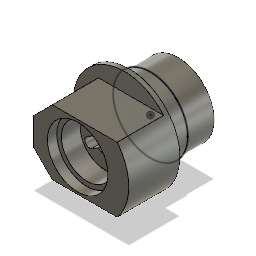
912-002_SpanDriver (Autodesk Fusion 360 design; units mm, degrees)
Autodesk Fusion 360 part; units mm, degrees
sketch "Sketch1" plane through (0, 0, 0) normal (0, 0, 1) x (1, 0, 0)
  circle A0 centre (0, 0) radius 3.875
  circle A1 centre (0, 0) radius 2.6825 construction
  circle A2 centre (0, 0) radius 2.356 construction
  line L0 (0, 2.356) -> (0, 2.6825)
  line L1 (-0.3686, 2.327) -> (-0.4196, 2.6495)
  line L2 (-0.728, 2.2407) -> (-0.8289, 2.5512)
  line L3 (-1.0696, 2.0992) -> (-1.2178, 2.3901)
  line L4 (-1.3848, 1.906) -> (-1.5767, 2.1702)
  line L5 (-1.6659, 1.6659) -> (-1.8968, 1.8968)
  line L6 (-1.906, 1.3848) -> (-2.1702, 1.5767)
  line L7 (-2.0992, 1.0696) -> (-2.3901, 1.2178)
  line L8 (-2.2407, 0.728) -> (-2.5512, 0.8289)
  line L9 (-2.327, 0.3686) -> (-2.6495, 0.4196)
  line L10 (-2.356, 0) -> (-2.6825, 0)
  line L11 (-2.327, -0.3686) -> (-2.6495, -0.4196)
  line L12 (-2.2407, -0.728) -> (-2.5512, -0.8289)
  line L13 (-2.0992, -1.0696) -> (-2.3901, -1.2178)
  line L14 (-1.906, -1.3848) -> (-2.1702, -1.5767)
  line L15 (-1.6659, -1.6659) -> (-1.8968, -1.8968)
  line L16 (-1.3848, -1.906) -> (-1.5767, -2.1702)
  line L17 (-1.0696, -2.0992) -> (-1.2178, -2.3901)
  line L18 (-0.728, -2.2407) -> (-0.8289, -2.5512)
  line L19 (-0.3686, -2.327) -> (-0.4196, -2.6495)
  line L20 (0, -2.356) -> (0, -2.6825)
  line L21 (0.3686, -2.327) -> (0.4196, -2.6495)
  line L22 (0.728, -2.2407) -> (0.8289, -2.5512)
  line L23 (1.0696, -2.0992) -> (1.2178, -2.3901)
  line L24 (1.3848, -1.906) -> (1.5767, -2.1702)
  line L25 (1.6659, -1.6659) -> (1.8968, -1.8968)
  line L26 (1.906, -1.3848) -> (2.1702, -1.5767)
  line L27 (2.0992, -1.0696) -> (2.3901, -1.2178)
  line L28 (2.2407, -0.728) -> (2.5512, -0.8289)
  line L29 (2.327, -0.3686) -> (2.6495, -0.4196)
  line L30 (2.356, 0) -> (2.6825, 0)
  line L31 (2.327, 0.3686) -> (2.6495, 0.4196)
  line L32 (2.2407, 0.728) -> (2.5512, 0.8289)
  line L33 (2.0992, 1.0696) -> (2.3901, 1.2178)
  line L34 (1.906, 1.3848) -> (2.1702, 1.5767)
  line L35 (1.6659, 1.6659) -> (1.8968, 1.8968)
  line L36 (1.3848, 1.906) -> (1.5767, 2.1702)
  line L37 (1.0696, 2.0992) -> (1.2178, 2.3901)
  line L38 (0.728, 2.2407) -> (0.8289, 2.5512)
  line L39 (0.3686, 2.327) -> (0.4196, 2.6495)
  line L40 (0, 2.6825) -> (-0.3686, 2.327)
  line L41 (0, 2.6825) -> (0.3686, 2.327)
  line L42 (-0.8289, 2.5512) -> (-0.3686, 2.327)
  line L43 (-0.8289, 2.5512) -> (-1.0696, 2.0992)
  line L44 (-1.5767, 2.1702) -> (-1.0696, 2.0992)
  line L45 (-1.5767, 2.1702) -> (-1.6659, 1.6659)
  line L46 (-2.1702, 1.5767) -> (-1.6659, 1.6659)
  line L47 (-2.1702, 1.5767) -> (-2.0992, 1.0696)
  line L48 (-2.5512, 0.8289) -> (-2.0992, 1.0696)
  line L49 (-2.5512, 0.8289) -> (-2.327, 0.3686)
  line L50 (-2.6825, 0) -> (-2.327, 0.3686)
  line L51 (-2.6825, 0) -> (-2.327, -0.3686)
  line L52 (-2.5512, -0.8289) -> (-2.327, -0.3686)
  line L53 (-2.5512, -0.8289) -> (-2.0992, -1.0696)
  line L54 (-2.1702, -1.5767) -> (-2.0992, -1.0696)
  line L55 (-2.1702, -1.5767) -> (-1.6659, -1.6659)
  line L56 (-1.5767, -2.1702) -> (-1.6659, -1.6659)
  line L57 (-1.5767, -2.1702) -> (-1.0696, -2.0992)
  line L58 (-0.8289, -2.5512) -> (-1.0696, -2.0992)
  line L59 (-0.8289, -2.5512) -> (-0.3686, -2.327)
  line L60 (0, -2.6825) -> (-0.3686, -2.327)
  line L61 (0, -2.6825) -> (0.3686, -2.327)
  line L62 (0.8289, -2.5512) -> (0.3686, -2.327)
  line L63 (0.8289, -2.5512) -> (1.0696, -2.0992)
  line L64 (1.5767, -2.1702) -> (1.0696, -2.0992)
  line L65 (1.5767, -2.1702) -> (1.6659, -1.6659)
  line L66 (2.1702, -1.5767) -> (1.6659, -1.6659)
  line L67 (2.1702, -1.5767) -> (2.0992, -1.0696)
  line L68 (2.5512, -0.8289) -> (2.0992, -1.0696)
  line L69 (2.5512, -0.8289) -> (2.327, -0.3686)
  line L70 (2.6825, 0) -> (2.327, -0.3686)
  line L71 (2.6825, 0) -> (2.327, 0.3686)
  line L72 (2.5512, 0.8289) -> (2.327, 0.3686)
  line L73 (2.5512, 0.8289) -> (2.0992, 1.0696)
  line L74 (2.1702, 1.5767) -> (2.0992, 1.0696)
  line L75 (2.1702, 1.5767) -> (1.6659, 1.6659)
  line L76 (1.5767, 2.1702) -> (1.6659, 1.6659)
  line L77 (1.5767, 2.1702) -> (1.0696, 2.0992)
  line L78 (0.8289, 2.5512) -> (1.0696, 2.0992)
  line L79 (0.8289, 2.5512) -> (0.3686, 2.327)
  dimension "d1" = 7.75
  dimension "d4" = 5.365
  dimension "d5" = 4.712
  dimension "d11" = 360
  dimension "d13" = 360
  constraint coincident A0.centre A1.centre
  constraint concentric A0 A1
  constraint concentric A1 A2
  constraint coincident A1 L0.end
  constraint vertical L0
  constraint coincident A2 L0.start
  measures "d1" diameter of A0
  measures "d4" diameter of A1
  measures "d5" diameter of A2
extrude "Extrude1" add sketch "Sketch1" along normal blind 3
sketch "Sketch2" plane through (0, 0, 3) normal (0, 0, 1) x (1, 0, 0)
  line L0 (1.0696, 2.0992) -> (1.5767, 2.1702)
  line L1 (1.5767, 2.1702) -> (1.6659, 1.6659)
  line L2 (1.6659, 1.6659) -> (2.1702, 1.5767)
  line L3 (2.1702, 1.5767) -> (2.0992, 1.0696)
  line L4 (2.0992, 1.0696) -> (2.5512, 0.8289)
  line L5 (2.5512, 0.8289) -> (2.327, 0.3686)
  line L6 (2.327, 0.3686) -> (2.6825, 0)
  line L7 (2.6825, 0) -> (2.327, -0.3686)
  line L8 (2.327, -0.3686) -> (2.5512, -0.8289)
  line L9 (2.5512, -0.8289) -> (2.0992, -1.0696)
  line L10 (2.0992, -1.0696) -> (2.1702, -1.5767)
  line L11 (2.1702, -1.5767) -> (1.6659, -1.6659)
  line L12 (1.6659, -1.6659) -> (1.5767, -2.1702)
  line L13 (1.5767, -2.1702) -> (1.0696, -2.0992)
  line L14 (1.0696, -2.0992) -> (0.8289, -2.5512)
  line L15 (0.8289, -2.5512) -> (0.3686, -2.327)
  line L16 (0.3686, -2.327) -> (0, -2.6825)
  line L17 (0, -2.6825) -> (-0.3686, -2.327)
  line L18 (-0.3686, -2.327) -> (-0.8289, -2.5512)
  line L19 (-0.8289, -2.5512) -> (-1.0696, -2.0992)
  line L20 (-1.0696, -2.0992) -> (-1.5767, -2.1702)
  line L21 (-1.5767, -2.1702) -> (-1.6659, -1.6659)
  line L22 (-1.6659, -1.6659) -> (-2.1702, -1.5767)
  line L23 (-2.1702, -1.5767) -> (-2.0992, -1.0696)
  line L24 (-2.0992, -1.0696) -> (-2.5512, -0.8289)
  line L25 (-2.5512, -0.8289) -> (-2.327, -0.3686)
  line L26 (-2.327, -0.3686) -> (-2.6825, 0)
  line L27 (-2.6825, 0) -> (-2.327, 0.3686)
  line L28 (-2.327, 0.3686) -> (-2.5512, 0.8289)
  line L29 (-2.5512, 0.8289) -> (-2.0992, 1.0696)
  line L30 (-2.0992, 1.0696) -> (-2.1702, 1.5767)
  line L31 (-2.1702, 1.5767) -> (-1.6659, 1.6659)
  line L32 (-1.6659, 1.6659) -> (-1.5767, 2.1702)
  line L33 (-1.5767, 2.1702) -> (-1.0696, 2.0992)
  line L34 (-1.0696, 2.0992) -> (-0.8289, 2.5512)
  line L35 (-0.8289, 2.5512) -> (-0.3686, 2.327)
  line L36 (-0.3686, 2.327) -> (0, 2.6825)
  line L37 (0, 2.6825) -> (0.3686, 2.327)
  line L38 (0.3686, 2.327) -> (0.8289, 2.5512)
  line L39 (0.8289, 2.5512) -> (1.0696, 2.0992)
  circle A0 centre (0, 0) radius 3.875
  circle A1 centre (0, 0) radius 4
  dimension "d16" = 8
  constraint coincident A0.centre A1.centre
  measures "d16" diameter of A1
extrude "Extrude2" add sketch "Sketch2" along normal blind 0.15 contours A0 | A1
sketch "Sketch3" plane through (0, 0, 3.15) normal (0, 0, 1) x (1, 0, 0)
  line L0 (0.3686, 2.327) -> (0.8289, 2.5512)
  line L1 (0.8289, 2.5512) -> (1.0696, 2.0992)
  line L2 (1.0696, 2.0992) -> (1.5767, 2.1702)
  line L3 (1.5767, 2.1702) -> (1.6659, 1.6659)
  line L4 (1.6659, 1.6659) -> (2.1702, 1.5767)
  line L5 (2.1702, 1.5767) -> (2.0992, 1.0696)
  line L6 (2.0992, 1.0696) -> (2.5512, 0.8289)
  line L7 (2.5512, 0.8289) -> (2.327, 0.3686)
  line L8 (2.327, 0.3686) -> (2.6825, 0)
  line L9 (2.6825, 0) -> (2.327, -0.3686)
  line L10 (2.327, -0.3686) -> (2.5512, -0.8289)
  line L11 (2.5512, -0.8289) -> (2.0992, -1.0696)
  line L12 (2.0992, -1.0696) -> (2.1702, -1.5767)
  line L13 (2.1702, -1.5767) -> (1.6659, -1.6659)
  line L14 (1.6659, -1.6659) -> (1.5767, -2.1702)
  line L15 (1.5767, -2.1702) -> (1.0696, -2.0992)
  line L16 (1.0696, -2.0992) -> (0.8289, -2.5512)
  line L17 (0.8289, -2.5512) -> (0.3686, -2.327)
  line L18 (0.3686, -2.327) -> (0, -2.6825)
  line L19 (0, -2.6825) -> (-0.3686, -2.327)
  line L20 (-0.3686, -2.327) -> (-0.8289, -2.5512)
  line L21 (-0.8289, -2.5512) -> (-1.0696, -2.0992)
  line L22 (-1.0696, -2.0992) -> (-1.5767, -2.1702)
  line L23 (-1.5767, -2.1702) -> (-1.6659, -1.6659)
  line L24 (-1.6659, -1.6659) -> (-2.1702, -1.5767)
  line L25 (-2.1702, -1.5767) -> (-2.0992, -1.0696)
  line L26 (-2.0992, -1.0696) -> (-2.5512, -0.8289)
  line L27 (-2.5512, -0.8289) -> (-2.327, -0.3686)
  line L28 (-2.327, -0.3686) -> (-2.6825, 0)
  line L29 (-2.6825, 0) -> (-2.327, 0.3686)
  line L30 (-2.327, 0.3686) -> (-2.5512, 0.8289)
  line L31 (-2.5512, 0.8289) -> (-2.0992, 1.0696)
  line L32 (-2.0992, 1.0696) -> (-2.1702, 1.5767)
  line L33 (-2.1702, 1.5767) -> (-1.6659, 1.6659)
  line L34 (-1.6659, 1.6659) -> (-1.5767, 2.1702)
  line L35 (-1.5767, 2.1702) -> (-1.0696, 2.0992)
  line L36 (-1.0696, 2.0992) -> (-0.8289, 2.5512)
  line L37 (-0.8289, 2.5512) -> (-0.3686, 2.327)
  line L38 (-0.3686, 2.327) -> (0, 2.6825)
  line L39 (0, 2.6825) -> (0.3686, 2.327)
  circle A0 centre (0, 0) radius 4
  line L40 (0, 0) -> (0, -0.9) construction
  line L41 (0, 0) -> (2, 0) construction
  line L42 (0, 0) -> (-1.7321, -1)
  line L43 (0, 0) -> (2, 0) construction
  circle A1 centre (0, 0) radius 1.3
  circle A2 centre (-1.7321, -1) radius 0.5
  line L44 (-1.9821, -0.567) -> (-1.2892, -0.167)
  line L45 (-1.4821, -1.433) -> (-0.2572, -1.433) construction
  line L46 (-1.4821, -1.433) -> (-0.7892, -1.033)
  dimension "d54" = 2
  dimension "d55" = 1
  dimension "d63" = 60
  constraint coincident A0.centre L40.start
  constraint vertical L40
  constraint horizontal L41
  constraint horizontal L43
  constraint coincident L42.end A2.centre
  constraint coincident A2 L44.start
  constraint coincident A1 L44.end
  constraint tangent A2 L44
  constraint horizontal L45
  constraint coincident A2 L45.start
  constraint parallel L44 L46
  constraint parallel L42 L44
  constraint tangent A2 L46
  constraint coincident A1 L46.end
  measures "d54" distance of A0.centre L42.end
  measures "d55" diameter of A2
  measures "d63" angle of L40 L42
extrude "Extrude8" add sketch "Sketch3" along normal blind 5 contours L25 L26 A2 | L25 L26 A2 | L42 A1 A2 L44 | L42 A1 A2 L46 | A1
extrude "Extrude3" add sketch "Sketch3" along normal blind 2.175 contours L25 L26 A2 | A0 picked at (-2.181, -1.0867)
sketch "Sketch4" plane through (0, 0, 5.325) normal (0, 0, 1) x (1, 0, 0)
  circle A0 centre (0, 0) radius 4
  circle A1 centre (0, 0) radius 5.5
  line L0 (-2.1702, -1.5767) -> (-2.1316, -1.3007)
  line L1 (-2.232, -0.9989) -> (-2.5512, -0.8289)
  arc A2 (-2.232, -0.9989) -> (-2.1316, -1.3007) centre (-1.7321, -1) ccw
  line L2 (-1.6659, -1.6659) -> (-2.1702, -1.5767)
  line L3 (-2.5512, -0.8289) -> (-2.327, -0.3686)
  line L4 (-2.327, -0.3686) -> (-2.6825, 0)
  line L5 (-2.6825, 0) -> (-2.327, 0.3686)
  line L6 (-2.327, 0.3686) -> (-2.5512, 0.8289)
  line L7 (-2.5512, 0.8289) -> (-2.0992, 1.0696)
  line L8 (-2.0992, 1.0696) -> (-2.1702, 1.5767)
  line L9 (-2.1702, 1.5767) -> (-1.6659, 1.6659)
  line L10 (-1.6659, 1.6659) -> (-1.5767, 2.1702)
  line L11 (-1.5767, 2.1702) -> (-1.0696, 2.0992)
  line L12 (-1.0696, 2.0992) -> (-0.8289, 2.5512)
  line L13 (-0.8289, 2.5512) -> (-0.3686, 2.327)
  line L14 (-0.3686, 2.327) -> (0, 2.6825)
  line L15 (0, 2.6825) -> (0.3686, 2.327)
  line L16 (0.3686, 2.327) -> (0.8289, 2.5512)
  line L17 (0.8289, 2.5512) -> (1.0696, 2.0992)
  line L18 (1.0696, 2.0992) -> (1.5767, 2.1702)
  line L19 (1.5767, 2.1702) -> (1.6659, 1.6659)
  line L20 (1.6659, 1.6659) -> (2.1702, 1.5767)
  line L21 (2.1702, 1.5767) -> (2.0992, 1.0696)
  line L22 (2.0992, 1.0696) -> (2.5512, 0.8289)
  line L23 (2.5512, 0.8289) -> (2.327, 0.3686)
  line L24 (2.327, 0.3686) -> (2.6825, 0)
  line L25 (2.6825, 0) -> (2.327, -0.3686)
  line L26 (2.327, -0.3686) -> (2.5512, -0.8289)
  line L27 (2.5512, -0.8289) -> (2.0992, -1.0696)
  line L28 (2.0992, -1.0696) -> (2.1702, -1.5767)
  line L29 (2.1702, -1.5767) -> (1.6659, -1.6659)
  line L30 (1.6659, -1.6659) -> (1.5767, -2.1702)
  line L31 (1.5767, -2.1702) -> (1.0696, -2.0992)
  line L32 (1.0696, -2.0992) -> (0.8289, -2.5512)
  line L33 (0.8289, -2.5512) -> (0.3686, -2.327)
  line L34 (0.3686, -2.327) -> (0, -2.6825)
  line L35 (0, -2.6825) -> (-0.3686, -2.327)
  line L36 (-0.3686, -2.327) -> (-0.8289, -2.5512)
  line L37 (-0.8289, -2.5512) -> (-1.0696, -2.0992)
  line L38 (-1.0696, -2.0992) -> (-1.5767, -2.1702)
  line L39 (-1.5767, -2.1702) -> (-1.6659, -1.6659)
  dimension "d24" = 11
  measures "d24" diameter of A1
extrude "Extrude4" add sketch "Sketch4" along normal blind 0.5 contours A0 | A1 | L0 L1 A2 L2 L3 L4 L5 L6 L7 L8 L9 L10 L11 L12 L13 L14 L15 L16 L17 L18 L19 L20 L21 L22 L23 L24 L25 L26 L27 L28 L29 L30 L31 L32 L33 L34 L35 L36 L37 L38 L39
sketch "Sketch5" plane through (0, 0, 5.825) normal (0, 0, 1) x (1, 0, 0)
  circle A0 centre (0, 0) radius 5.5
  circle A1 centre (0, 0) radius 2.75
  circle A2 centre (0, 0) radius 5.5
  arc A3 (4.2426, -3.5) -> (1.0617, 5.3966) centre (0, 0) ccw
  line L0 (-2.7574, -3.5) -> (-4.7574, -1.5)
  line L1 (-4.7574, -1.5) -> (-4.7574, 1.5)
  line L2 (-4.7574, 1.5) -> (-2.7574, 3.5)
  line L3 (-2.7574, 3.5) -> (4.2426, 3.5)
  line L4 (-2.7574, -3.5) -> (4.2426, -3.5)
  arc A4 (-1.9821, -0.567) -> (-1.4821, -1.433) centre (-1.7321, -1) ccw
  line L5 (-1.9821, -0.567) -> (-1.2892, -0.167)
  arc A5 (-0.7892, -1.033) -> (-1.2892, -0.167) centre (0, 0) ccw
  line L6 (-0.7892, -1.033) -> (-1.4821, -1.433)
  dimension "d28" = 5.5
  dimension "d41" = 2
  dimension "d43" = 7
  dimension "d45" = 2
  dimension "d46" = 2
  dimension "d48" = 2
  dimension "d49" = 3
  dimension "d50" = 1.5
  constraint coincident A0.centre A1.centre
  constraint coincident A2 A3.start
  constraint coincident A2 A3.end
  constraint horizontal L3
  constraint coincident A2 L3.end
  constraint coincident A3 L3.end
  constraint horizontal L4
  constraint vertical L1
  measures "d28" diameter of A1
  measures "d41" distance of L2.end L1
  measures "d43" distance of L2.end L3.end
  measures "d45" vertical distance of L2.end L1.end
  measures "d46" vertical distance of L0.start L0.end
  measures "d48" horizontal distance of L0.start L0.end
  measures "d49" distance of L0.end L1.end
  measures "d50" vertical distance of A0.centre L1.end
extrude "Extrude5" add sketch "Sketch5" along normal blind 2 contours A0 A2 A3 L0 L1 L2 L3 L4 | A1 | A4 L5 A5 L6 picked at (-4.0882, 0)
sketch "Sketch6" plane through (0, 0, 7.825) normal (0, 0, 1) x (1, 0, 0)
  circle A0 centre (0, 0) radius 2.75
  line L0 (-4.7574, -1.5) -> (-2.7574, -3.5)
  line L1 (-2.7574, -3.5) -> (4.2426, -3.5)
  arc A1 (4.2426, -3.5) -> (4.2426, 3.5) centre (0, 0) ccw
  line L2 (4.2426, 3.5) -> (-2.7574, 3.5)
  line L3 (-2.7574, 3.5) -> (-4.7574, 1.5)
  line L4 (-4.7574, 1.5) -> (-4.7574, -1.5)
  arc A2 (-0.7892, -1.033) -> (-1.2892, -0.167) centre (0, 0) ccw
  arc A3 (-1.9821, -0.567) -> (-1.4821, -1.433) centre (-1.7321, -1) ccw
  line L5 (-1.9821, -0.567) -> (-1.2892, -0.167)
  line L6 (-0.7892, -1.033) -> (-1.4821, -1.433)
  dimension "d35" = 5.5
  constraint coincident A0.centre A1.centre
  measures "d35" diameter of A0
extrude "Extrude6" add sketch "Sketch6" along normal blind 3 contours L0 L1 A1 L2 L3 L4
sketch "Sketch7" plane through (0, 0, 10.825) normal (0, 0, 1) x (1, 0, 0)
  circle A0 centre (0, 0) radius 2.75
  circle A1 centre (0, 0) radius 3.25
  line L0 (-4.7574, 1.5) -> (-4.7574, -1.5)
  line L1 (-4.7574, -1.5) -> (-2.7574, -3.5)
  line L2 (-2.7574, -3.5) -> (4.2426, -3.5)
  arc A2 (4.2426, -3.5) -> (4.2426, 3.5) centre (0, 0) ccw
  line L3 (4.2426, 3.5) -> (-2.7574, 3.5)
  line L4 (-2.7574, 3.5) -> (-4.7574, 1.5)
  dimension "d38" = 6.5
  constraint coincident A0.centre A1.centre
  measures "d38" diameter of A1
extrude "Extrude7" cut sketch "Sketch7" against normal blind 1 contours A1
extrude "Extrude9" cut 1 faces at (-0.3747, -0.1058, 8.15) along direction (0, 0, -1) blind 5
extrude "Extrude10" cut 1 faces at (-2.181, -1.0867, 3.15) along direction (0, 0, -1) blind 3.15
equation "d22 = 2.325 mm - 0.15 mm"
